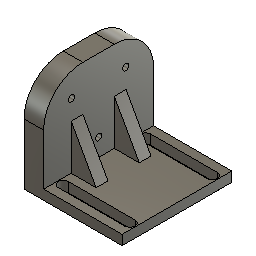
RollersSupport4 (Autodesk Fusion 360 design; units mm, degrees)
Autodesk Fusion 360 part; units mm, degrees
note: some values were not read from the file. Chosen so that the rebuilt part matches the saved one: a direction; that a step has no effect.
sketch "Sketch1" plane through (0, 0, 0) normal (0, 1, 0) x (1, 0, 0)
  line L0 (0, 0) -> (50, 0)
  line L1 (50, 0) -> (50, -56)
  line L2 (50, -56) -> (0, -56)
  line L3 (0, -56) -> (0, 0)
  line L4 (0, -28) -> (50, -28)
  line L5 (13, -4.35) -> (47, -4.35)
  line L6 (13, -9.65) -> (47, -9.65)
  arc A0 (13, -4.35) -> (13, -9.65) centre (13, -7) ccw
  arc A1 (47, -9.65) -> (47, -4.35) centre (47, -7) ccw
  line L7 (13, -46.35) -> (47, -46.35)
  arc A2 (13, -46.35) -> (13, -51.65) centre (13, -49) ccw
  line L8 (13, -51.65) -> (47, -51.65)
  arc A3 (47, -51.65) -> (47, -46.35) centre (47, -49) ccw
  dimension "d1" = 50
  dimension "d2" = 56
  dimension "d4" = 5.3
  dimension "d6" = 21
  dimension "d7" = 13
  dimension "d8" = 5.3
  dimension "d9" = 3
  constraint horizontal L0
  constraint vertical L1
  constraint horizontal L2
  constraint vertical L3
  constraint coincident L0.start L3.end
  constraint midpoint L3 L4.start
  constraint midpoint L1 L4.end
  constraint tangent L5 A1
  constraint tangent L5 A0
  constraint coincident L6.start A0
  constraint tangent L6 A1
  constraint tangent L6 A0
  constraint coincident L6 A0.end
  constraint symmetric L4 L5.start A2.end
  constraint symmetric L4 L5.end L8.end
  constraint symmetric L4 L6.start L7.start
  constraint symmetric L4 L6.end L7.end
  constraint symmetric L4 A0 A2
  constraint symmetric L4 A1 A3
  constraint parallel L4 L6
  measures "d1" distance of L0.start L0.end
  measures "d2" distance of L0.start L2.end
  measures "d4" diameter of A0
  measures "d6" distance of L4 A0.centre
  measures "d7" distance of L3 A0.centre
  measures "d8" diameter of A1
  measures "d9" distance of L1 A1.centre
extrude "Extrude1" add sketch "Sketch1" along normal blind 5
sketch "Sketch2" plane through (0, 5, 0) normal (0, 1, 0) x (-1, 0, 0)
  arc A0 (-13, 4.35) -> (-13, 9.65) centre (-13, 7) ccw
  line L0 (-13, 4.35) -> (-47, 4.35)
  arc A1 (-47, 9.65) -> (-47, 4.35) centre (-47, 7) ccw
  line L1 (-47, 9.65) -> (-13, 9.65)
  arc A2 (-13, 46.35) -> (-13, 51.65) centre (-13, 49) ccw
  line L2 (-13, 46.35) -> (-47, 46.35)
  arc A3 (-47, 51.65) -> (-47, 46.35) centre (-47, 49) ccw
  line L3 (-47, 51.65) -> (-13, 51.65)
  line L4 (0, 56) -> (-50, 56)
  line L5 (-50, 56) -> (-50, 0)
  line L6 (-50, 0) -> (0, 0)
  line L7 (0, 0) -> (0, 56)
  line L8 (-10, 0) -> (-10, 56)
  dimension "d12" = 10
  constraint coincident L6 L8.start
  constraint coincident L4 L8.end
  constraint perpendicular L4 L8
  measures "d12" distance of L7 L8
extrude "Extrude2" add sketch "Sketch2" along normal blind 46 contours L4 L6 L7 L8
extrude "Extrude3" [no effect]
sketch "Sketch4" plane through (0, 0, 0) normal (-1, 0, 0) x (0, 0, 1)
  line L0 (0, 0) -> (56, 0)
  line L1 (56, 0) -> (56, 51)
  line L2 (56, 51) -> (0, 51)
  line L3 (0, 51) -> (0, 0)
  circle A0 centre (28, 30) radius 13
  line L4 (28, 51) -> (28, 43)
  line L5 (28, 17) -> (28, 0)
  dimension "d19" = 26
  dimension "d20" = 30
  constraint midpoint L2 L4.start
  constraint midpoint L0 L5.end
  constraint coincident A0 L4.end
  constraint coincident A0 L5.start
  constraint collinear L4 L5
  constraint coincident A0.centre L4
  measures "d19" diameter of A0
  measures "d20" distance of L0 A0.centre
extrude "Extrude4" cut sketch "Sketch4" against normal blind 6.5 contours A0
sketch "Sketch5" plane through (0, 0, 0) normal (-1, 0, 0) x (0, 0, 1)
  circle A0 centre (28, 30) radius 13
  line L0 (0, 0) -> (56, 0)
  line L1 (56, 0) -> (56, 51)
  line L2 (56, 51) -> (0, 51)
  line L3 (0, 51) -> (0, 0)
  circle A1 centre (28, 14) radius 1.6
  line L4 (28, 30) -> (56, 13.8342)
  line L5 (28, 30) -> (60.3316, 30) construction
  line L6 (28, 30) -> (0, 13.8342)
  circle A2 centre (14.1436, 38) radius 1.6
  circle A3 centre (41.8564, 38) radius 1.6
  dimension "d23" = 3.2
  dimension "d24" = 16
  dimension "d25" = 30
  constraint horizontal L5
  constraint coincident A0.centre L4.start
  constraint coincident L1 L4.end
  constraint coincident L3 L6.end
  constraint symmetric A1 L6 A2
  constraint symmetric A1 L4 A3
  measures "d23" diameter of A1
  measures "d24" distance of A0.centre A1.centre
  measures "d25" angle of L4 L5
extrude "Extrude5" cut sketch "Sketch5" against normal blind 10 contours A1 | A2 | A3
ref_plane "WorkPlane1" through (25, 25.5, 20) normal (0, 0, -1) x (-1, 0, 0)
sketch "Sketch6" plane through (25, 25.5, 20) normal (0, 0, -1) x (1, 0, 0)
ref_plane "WorkPlane3" through (0, 0, 17) normal (0, 0, 1) x (1, 0, 0)
sketch "Sketch7" plane through (0, 0, 17) normal (0, 0, 1) x (1, 0, 0)
sketch "Sketch8" plane through (0, 0, 17) normal (0, 0, 1) x (1, 0, 0)
  line L0 (10, 5) -> (10, 51)
  line L1 (50, 5) -> (10, 5)
  line L2 (10, 28) -> (22.7682, 5)
  constraint midpoint L0 L2.start
  constraint coincident L1 L2.end
rib "Rib1" add thickness 6 on both sides direction (-0.874312, -0.485363, 0) up to next extending the curves path "Sketch8" along L2
pattern_linear "R-Pattern1" count 2 spacing 22 along (0, 0, 1) of "Rib1"
fillet "Fillet1" radius 20 1 edges at (5, 51, 56)
fillet "Fillet2" radius 20 1 edges at (5, 51, 0)
sketch "Sketch9" plane through (0, 0, 0) normal (-1, 0, 0) x (0, 0, 1)
  arc A0 (20, 51) -> (0, 31) centre (20, 31) ccw
  line L0 (0, 31) -> (0, 0)
  line L1 (0, 0) -> (56, 0)
  line L2 (56, 0) -> (56, 31)
  arc A1 (56, 31) -> (36, 51) centre (36, 31) ccw
  line L3 (36, 51) -> (20, 51)
  circle A2 centre (41.8564, 38) radius 1.6
  circle A3 centre (28, 30) radius 13
  circle A4 centre (14.1436, 38) radius 1.6
  circle A5 centre (28, 14) radius 1.6
  line L4 (45.3383, 2) -> (45.3383, 4.3943)
  line L5 (45.3383, 4.3943) -> (41, 4.3943)
  line L6 (41, 4.3943) -> (41, 5.5198)
  line L7 (41, 5.5198) -> (45.5634, 12)
  line L8 (45.5634, 12) -> (46.5662, 12)
  line L9 (46.5662, 12) -> (46.5662, 5.5198)
  line L10 (46.5662, 5.5198) -> (47.9168, 5.5198)
  line L11 (47.9168, 5.5198) -> (47.9168, 4.3943)
  line L12 (47.9168, 4.3943) -> (46.5662, 4.3943)
  line L13 (46.5662, 4.3943) -> (46.5662, 2)
  line L14 (46.5662, 2) -> (45.3383, 2)
  line L15 (45.3383, 5.5198) -> (45.3383, 10.0286)
  line L16 (45.3383, 10.0286) -> (42.2074, 5.5198)
  line L17 (42.2074, 5.5198) -> (45.3383, 5.5198)
extrude "Extrude6" cut sketch "Sketch9" against normal blind 1 contours L4 L5 L6 L7 L8 L9 L10 L11 L12 L13 L14
fillet "Fillet3" radius 1.5 1 edges at (0, 34.701, 15.8797)
